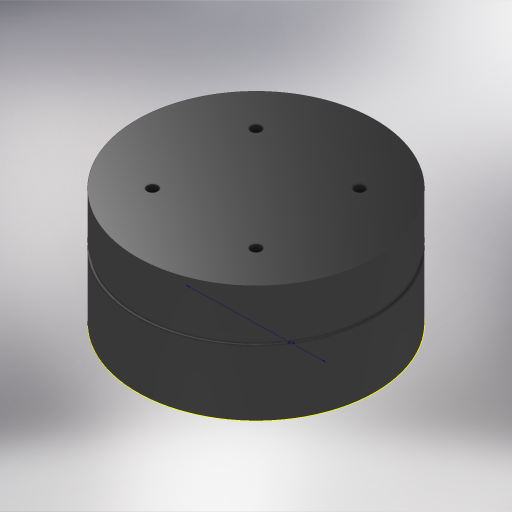
# Autodesk Inventor part: motor
Saved by Autodesk Inventor 2024.3 (Build 283343000, 343)
## iProperties
Created: 2024-06-05
Part Number: motor
Material: Generic
Document SubType Name: Modeling
Designer: danie
Density: 1 g/cm^3
Appearance: Default
Author: danie
Autodesk Inventor part; units mm, degrees
ref_plane "YZ Plane" through (0, 0, 0) normal (1, 0, 0) x (0, 1, 0)
ref_plane "XZ Plane" through (0, 0, 0) normal (0, 1, 0) x (-1, 0, 0)
ref_plane "XY Plane" through (0, 0, 0) normal (0, 0, 1) x (1, 0, 0)
sketch "Sketch1" plane through (0, 0, 0) normal (0, 1, 0) x (-1, 0, 0)
  circle A0 centre (0, 0) radius 34.5
  dimension "d0" = 69
  constraints: 1 centre point, 1 coincident
  measures "d0" diameter of A0
extrude "Extrusion1" add sketch "Sketch1" along normal blind 33.9
sketch "Sketch2" plane through (0, 33.9, 0) normal (0, 1, 0) x (1, 0, 0)
  circle A0 centre (0, 0) radius 34.5 projected
  line L0 (-15, -15) -> (15, -15)
  line L1 (15, -15) -> (15, 15)
  line L2 (15, 15) -> (-15, 15)
  line L3 (-15, 15) -> (-15, -15)
  line L4 (-15, -15) -> (15, 15) construction
  line L5 (15, -15) -> (-15, 15) construction
  circle A1 centre (-15, 15) radius 1.5
  circle A2 centre (15, 15) radius 1.5
  circle A3 centre (-15, -15) radius 1.5
  circle A4 centre (15, -15) radius 1.5
  dimension "d3" = 30
  dimension "d4" = 30
  dimension "d5" = 3
  dimension "d6" = 3
  dimension "d7" = 3
  dimension "d8" = 3
  constraints: 12 end point, 4 centre point, 4 coincident, 2 midpoint, 2 parallel, 1 horizontal, 1 perpendicular
  measures "d3" distance between parallel lines of L2 L0
  measures "d4" distance between parallel lines of L3 L1
  measures "d5" diameter of A1
  measures "d6" diameter of A2
  measures "d7" diameter of A3
  measures "d8" diameter of A4
hole "Hole1" at (-15, 33.9, 15) at (15, 33.9, 15) at (-15, 33.9, -15) at (15, 33.9, -15) direction (0, -1, 0) diameter 3 depth 10.4
sketch "Sketch3" plane through (0, 0, 0) normal (0, -1, 0) x (1, 0, 0)
  circle A0 centre (0, 0) radius 34.5 projected
  circle A1 centre (0, 0) radius 6.35
  dimension "d16" = 12.7
  constraints: 1 centre point, 1 coincident
  measures "d16" diameter of A1
extrude "Extrusion2" cut sketch "Sketch3" against normal blind 20 contours A1
ref_plane "Work Plane1" through (0, 20, 0) normal (0, -1, 0) x (1, 0, 0)
sketch "Sketch4" plane through (0, 20, 0) normal (0, -1, 0) x (1, 0, 0)
  circle A0 centre (0, 0) radius 6.35 projected
  circle A1 centre (0, 0) radius 34.5 projected
  circle A2 centre (0, 0) radius 34
  dimension "d20" = 68
  constraints: 1 centre point, 1 coincident
  measures "d20" diameter of A2
extrude "Extrusion3" cut sketch "Sketch4" along normal mid plane 2 contours A1
sketch "Sketch5" plane through (0, 0, 0) normal (0, -1, 0) x (1, 0, 0)
  circle A0 centre (0, 0) radius 6.35 projected
  circle A1 centre (0, 0) radius 34.5 projected
  circle A2 centre (0, 0) radius 12.5
  line L0 (0, -1) -> (0, -12.5)
  circle A3 centre (0, -12.5) radius 2
  circle A4 centre (12.5, 0) radius 2
  circle A5 centre (0, 12.5) radius 2
  circle A6 centre (-12.5, 0) radius 2
  dimension "d23" = 25
  dimension "d24" = 4
  dimension "d27" = 360
  constraints: 5 coincident, 4 centre point, 2 end point, 1 vertical, 1 vertical alignment, 15 other
  measures "d24" diameter of A3
hole "Hole2" at (0, 0, -12.5) at (12.5, 0, 0) at (0, 0, 12.5) at (-12.5, 0, 0) direction (0, 1, 0) diameter 3 depth 3.5
sketch "Sketch6" plane through (0, 0, 0) normal (0, -1, 0) x (1, 0, 0)
  line L0 (-63, 66) -> (64.0177, 66) construction
  line L1 (64.0177, 66) -> (64.0177, -63.3993) construction
  line L2 (64.0177, -63.3993) -> (-63, -63.3993) construction
  line L3 (-63, -63.3993) -> (-63, 66) construction
  point P0 (0, 0)
  constraints: 2 other
decal "Decal1"
sketch "Sketch8" plane through (0, 0, 0) normal (0, -1, 0) x (1, 0, 0)
  circle A0 centre (-12.5, 0) radius 1.5 projected
  circle A1 centre (0, 12.5) radius 1.5 projected
  circle A2 centre (12.5, 0) radius 1.5 projected
  circle A3 centre (0, -12.5) radius 1.5 projected
  circle A4 centre (0, 0) radius 6.35 projected
  circle A5 centre (0, 0) radius 34.5 projected
  circle A6 centre (0, 0) radius 12.5
  circle A7 centre (0, 0) radius 19.8
  dimension "d39" = 39.6
  constraints: 2 coincident, 1 centre point, 1 horizontal alignment, 2 other
  measures "d39" diameter of A7
body "Solid1"
